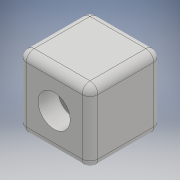
# Autodesk Inventor part: Hombro
Saved by Autodesk Inventor 2017 (Build 210142000, 142)
## iProperties
Part Number: Hombro
Material: Genérico
Document SubType Name: Modeling
Designer: HOME
Density: 1 g/cm^3
Appearance: Valor por defecto
Author: HOME
Autodesk Inventor part; units mm, degrees
ref_plane "YZ Plane" through (0, 0, 0) normal (1, 0, 0) x (0, 1, 0)
ref_plane "XZ Plane" through (0, 0, 0) normal (0, 1, 0) x (-1, 0, 0)
ref_plane "XY Plane" through (0, 0, 0) normal (0, 0, 1) x (1, 0, 0)
sketch "Boceto1" plane through (0, 0, 0) normal (0, 0, 1) x (1, 0, 0)
  line L0 (9, 9) -> (-9, 9)
  line L1 (-9, 9) -> (-9, -9)
  line L2 (-9, -9) -> (9, -9)
  line L3 (9, -9) -> (9, 9)
  line L4 (9, 9) -> (-9, -9) construction
  line L5 (-9, 9) -> (9, -9) construction
  point P0 (0, 0)
  dimension "d0" = 18
  constraints: 12 end point, 4 perpendicular, 2 midpoint, 1 vertical
  measures "d0" distance of L0.end L1.end
extrude "Extrusión1" add sketch "Boceto1" along normal blind 18
fillet "Empalme1" radius 2 12 edges at (9, 0, 0) (9, 9, 9) (9, 0, 18) (9, -9, 9) (0, -9, 0) (0, -9, 18) (-9, -9, 9) (-9, 0, 0) (-9, 0, 18) (-9, 9, 9) (0, 9, 0) (0, 9, 18)
sketch "Boceto2" plane through (0, 0, 0) normal (0, 0, -1) x (-1, 0, 0)
  circle A0 centre (0, 0) radius 4.025
  dimension "d4" = 8.05
  constraints: 1 centre point, 1 coincident
  measures "d4" diameter of A0
extrude "Extrusión2" cut sketch "Boceto2" against normal blind 5
sketch "Boceto3" plane through (-7, -9, 2) normal (0, -1, 0) x (1, 0, 0)
  circle A0 centre (7, 7) radius 4.025
  line L0 (14, 0) -> (0, 0) projected
  line L1 (0, 0) -> (0, 14) projected
  point P0 (7, -2)
  dimension "d7" = 8.05
  dimension "d8" = 7
  dimension "d9" = 7
  constraints: 1 centre point
  measures "d7" diameter of A0
  measures "d8" distance from line of L0 A0.centre
  measures "d9" distance from line of L1 A0.centre
extrude "Extrusión3" cut sketch "Boceto3" against normal blind 5
